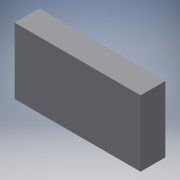
# Autodesk Inventor part: SuporteGuiasCabeçasAquecimento
Saved by Autodesk Inventor 2018 (Build 220112000, 112)
## iProperties
Created: 2018-07-23
Part Number: SuporteGuiasCabeçasAquecimento
Material: Genérico
Document SubType Name: Modeling
Designer: Usuario
Density: 1 g/cm^3
Appearance: Padrão
Author: Usuario
Autodesk Inventor part; units mm, degrees
ref_plane "YZ Plane" through (0, 0, 0) normal (1, 0, 0) x (0, 1, 0)
ref_plane "XZ Plane" through (0, 0, 0) normal (0, 1, 0) x (-1, 0, 0)
ref_plane "XY Plane" through (0, 0, 0) normal (0, 0, 1) x (1, 0, 0)
sketch "Esboço1" plane through (0, 0, 0) normal (0, 0, 1) x (1, 0, 0)
  line L0 (-34.4331, 106.027) -> (41.7669, 106.027)
  line L1 (41.7669, 106.027) -> (41.7669, 91.027)
  line L2 (41.7669, 91.027) -> (-34.4331, 91.027)
  line L3 (-34.4331, 91.027) -> (-34.4331, 106.027)
  point P0 (0, 0)
  dimension "d0" = 76.2
  dimension "d1" = 15
  constraints: 8 end point, 2 parallel, 1 horizontal, 1 perpendicular
  measures "d0" distance of L1.end L2.end
  measures "d1" distance of L0.end L1.end
extrude "Extrusão1" add sketch "Esboço1" along normal blind 40
sketch "Esboço2" plane through (-34.4331, 106.027, 0) normal (0, 1, 0) x (1, 0, 0)
  line L0 (76.2, 0) -> (76.2, -40) projected
  line L1 (76.2, -20) -> (0, -20)
  line L2 (0, 0) -> (0, -40) projected
  line L3 (0, 0) -> (76.2, 0) projected
  line L4 (38.1, -40) -> (38.1, 0)
  circle A0 centre (59.1, -20) radius 6.7139
  circle A1 centre (17.1, -20) radius 6.7459
  point P0 (34.4331, 0)
  dimension "d4" = 20
  dimension "d5" = 21
  dimension "d6" = 21
  constraints: 4 end point, 3 midpoint, 2 centre point, 2 point on line, 1 horizontal
  measures "d4" distance between parallel lines of L3 L1
  measures "d5" distance from line of A0.centre L4
  measures "d6" distance from line of L4 A1.centre
hole "Furo1" at (24.6669, 106.027, 20) at (-17.3331, 106.027, 20) direction (0, -1, 0) diameter 12 depth 7.5
sketch "Esboço3" plane through (0, 0, 0) normal (0, 0, -1) x (-1, 0, 0)
  line L0 (-41.7669, 91.027) -> (-41.7669, 106.027) construction
  line L1 (-41.7669, 98.527) -> (34.4331, 98.527) construction
  line L2 (34.4331, 106.027) -> (34.4331, 91.027) construction
  line L3 (-41.7669, 106.027) -> (34.4331, 106.027) construction
  line L4 (-32.2419, 106.027) -> (-32.2419, 91.027) construction
  line L5 (24.9081, 106.027) -> (24.9081, 91.027) construction
  line L6 (-3.6669, 106.027) -> (-3.6669, 91.027) construction
  line L7 (-18.6669, 98.527) -> (-30.6669, 98.527) construction
  circle A0 centre (-32.2419, 98.527) radius 2 construction
  circle A1 centre (-3.6669, 98.527) radius 2 construction
  line L8 (23.3331, 98.527) -> (11.3331, 98.527) construction
  circle A2 centre (24.9081, 98.527) radius 2 construction
  point P0 (0, 0)
  dimension "d14" = 9.525
  dimension "d15" = 9.525
  dimension "d16" = 38.1
  dimension "d17" = 4
  dimension "d18" = 4
  dimension "d19" = 4
  constraints: 8 end point, 6 midpoint, 4 point on line, 3 centre point, 3 vertical
  measures "d14" distance between parallel lines of L5 L2
  measures "d15" distance between parallel lines of L0 L4
  measures "d16" distance between parallel lines of L0 L6
  measures "d17" diameter of A0
  measures "d18" diameter of A1
  measures "d19" diameter of A2
hole "Furo2" at (32.2419, 98.527, 0) at (3.6669, 98.527, 0) at (-24.9081, 98.527, 0) direction (0, 0, 1) diameter 3.242 depth 12 thread size "M4x0.7" class "6H" standard "ANSI Metric M Profile"
equation "\"d4\" = 0.5 * d2"
equation "\"d6\" = d5"
equation "\"d12\" = 0.5 * d1"
equation "\"d14\" = d15"
equation "\"d15\" = 0.125 * d0"
equation "\"d16\" = 0.5 * d0"
equation "\"d2\" = 40"
